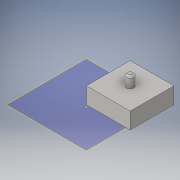
# Autodesk Inventor part: Elektrodenhaltr3.0
Saved by Autodesk Inventor 2016 (Build 200138000, 138)
## iProperties
Created: 2016-08-09
Part Number: Elektrodenhaltr3.0
Material: Generisch
Document SubType Name: Modeling
Designer: arminius
Density: 1 g/cm^3
Appearance: Vorgabe
Author: arminius
Autodesk Inventor part; units mm, degrees
ref_plane "YZ Plane" through (0, 0, 0) normal (1, 0, 0) x (0, 1, 0)
ref_plane "XZ Plane" through (0, 0, 0) normal (0, 1, 0) x (-1, 0, 0)
ref_plane "XY Plane" through (0, 0, 0) normal (0, 0, 1) x (1, 0, 0)
sketch "Skizze1" plane through (0, 0, 0) normal (0, 0, 1) x (1, 0, 0)
  line L0 (0, 0) -> (12, 0)
  line L1 (12, 0) -> (12, 12)
  line L2 (12, 12) -> (0, 12)
  line L3 (0, 12) -> (0, 0)
  dimension "d0" = 12
  dimension "d1" = 12
  constraints: 8 end point, 2 parallel, 1 horizontal, 1 perpendicular
  measures "d0" distance between parallel lines of L0 L2
  measures "d1" distance between parallel lines of L3 L1
extrude "Extrusion1" add sketch "Skizze1" along normal blind 5
sketch "Skizze2" plane through (0, 0, 5) normal (0, 0, 1) x (1, 0, 0)
  circle A0 centre (6, 6) radius 1
  line L0 (12, 0) -> (12, 12) projected
  line L1 (0, 0) -> (12, 0) projected
  dimension "d4" = 6
  dimension "d5" = 6
  dimension "d6" = 2
  constraints: 1 centre point
  measures "d4" distance from line of L0 A0.centre
  measures "d5" distance from line of A0.centre L1
  measures "d6" diameter of A0
extrude "Extrusion2" add sketch "Skizze2" along normal blind 3
chamfer "Fase1" distance 0.5 angle 45 1 edges at (5, 6, 8)
sketch "Skizze3" plane through (0, 12, 0) normal (0, 1, 0) x (1, 0, 0)
  line L0 (0, 0) -> (12, 0) projected
  circle A0 centre (6, 0) radius 2.25
  dimension "d12" = 4.5
  constraints: 1 centre point, 1 midpoint
  measures "d12" diameter of A0
extrude "Extrusion3" cut sketch "Skizze3" against normal blind 4
sketch "Skizze4" plane through (0, 0, 0) normal (0, 0, -1) x (-1, 0, 0)
  circle A0 centre (-6, 6) radius 0.5 projected
  circle A1 centre (-6, 6) radius 5.4
  point P0 (0, 0)
  constraints: 1 centre point, 1 coincident
ref_plane "Arbeitsebene1" through (0, 0, 0.5) normal (0, 0, -1) x (-1, 0, 0)
sketch "Skizze5" plane through (0, 0, 0.5) normal (0, 0, -1) x (-1, 0, 0)
  circle A0 centre (-6, 6) radius 0.5 projected
  circle A1 centre (-6, 6) radius 3.55
  point P0 (0, 0)
  dimension "d18" = 7.1
  constraints: 1 centre point, 1 coincident
  measures "d18" diameter of A1
extrude "Extrusion5" cut sketch "Skizze5" against normal blind 2.7
sketch "Skizze6" plane through (0, 12, 5) normal (0, 1, 0) x (1, 0, 0)
  line L0 (12, 4.5) -> (0, 4.5)
  line L1 (0, 4.5) -> (0, 5)
  line L2 (0, 5) -> (12, 5)
  line L3 (12, 5) -> (12, 4.5)
  line L4 (0, 5) -> (0, 0) projected
  line L5 (3.75, 5) -> (0, 5) projected
  line L6 (12, 5) -> (12, 0) projected
  line L7 (3.8063, 4.5) -> (8.1937, 4.5) projected
  dimension "d24" = 0
  dimension "d25" = 0
  dimension "d26" = 0
  dimension "d27" = 0
  constraints: 8 end point, 2 parallel, 1 horizontal, 1 perpendicular
  measures "d24" distance between parallel lines of L4 L1
  measures "d25" distance between parallel lines of L5 L2
  measures "d26" distance between parallel lines of L6 L3
  measures "d27" distance between parallel lines of L7 L0
extrude "Extrusion6" cut sketch "Skizze6" against normal blind 20
fillet "Rundung1" radius 2 1 edges at (9.55, 6, 3.2)
